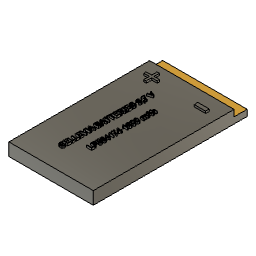
eBook_Reader (Autodesk Fusion 360 archive; units mm, degrees)
design "baterie"
Autodesk Fusion 360 part; units mm, degrees
sketch "Sketch1" plane through (0, 0, 0) normal (0, 0, 1) x (1, 0, 0)
  line L0 (0, 0) -> (42, 0)
  line L1 (42, 0) -> (42, 76.5)
  line L2 (42, 76.5) -> (0, 76.5)
  line L3 (0, 76.5) -> (0, 0)
  dimension "d1" = 42
  dimension "d2" = 76.5
  constraint horizontal L0
  constraint vertical L1
  constraint horizontal L2
  constraint vertical L3
  constraint coincident L0.start L3.end
  measures "d1" distance of L0.start L0.end
  measures "d2" distance of L0.start L2.end
extrude "Extrude1" add sketch "Sketch1" along normal blind 6.3
sketch "Sketch2" plane through (0, 0, 6.3) normal (0, 0, 1) x (-1, 0, 0)
  line L0 (0, -76.5) -> (0, 0)
  line L1 (0, 0) -> (-42, 0)
  line L2 (-42, 0) -> (-42, -76.5)
  line L3 (-42, -76.5) -> (0, -76.5)
  line L4 (0, -70) -> (-42, -70)
  constraint coincident L0 L4.start
  constraint coincident L2 L4.end
  constraint perpendicular L2 L4
extrude "Extrude2" cut sketch "Sketch2" against normal blind 3.2 contours L0 L2 L3 L4
sketch "Sketch3" plane through (0, 0, 6.3) normal (0, 0, 1) x (-1, 0, 0)
  line L0 (-42, -70) -> (0, -70)
  line L1 (0, -70) -> (0, 0)
  line L2 (0, 0) -> (-42, 0)
  line L3 (-42, 0) -> (-42, -70)
  line L4 (-5, -58) -> (-14, -58) construction
  line L5 (-14, -58) -> (-14, -66) construction
  line L6 (-14, -66) -> (-5, -66) construction
  line L7 (-5, -66) -> (-5, -58) construction
  dimension "d7" = 10
  text T0 "+\n" font "Arial" height 10 align left top in box 9 x 8 at (-5, -58) x (-1, 0) y (0, -1) spacing 1 kerned
extrude "Extrude3" add sketch "Sketch3" along normal blind 1 text T0
sketch "Sketch4" plane through (0, 0, 6.3) normal (0, 0, 1) x (-1, 0, 0)
  line L0 (-7.7217, -59.3902) -> (-7.7217, -62.1323)
  line L1 (-7.7217, -62.1323) -> (-5, -62.1323)
  line L2 (-5, -62.1323) -> (-5, -63.2783)
  line L3 (-5, -63.2783) -> (-7.7217, -63.2783)
  line L4 (-7.7217, -63.2783) -> (-7.7217, -66)
  line L5 (-7.7217, -66) -> (-8.8813, -66)
  line L6 (-8.8813, -66) -> (-8.8813, -63.2783)
  line L7 (-8.8813, -63.2783) -> (-11.603, -63.2783)
  line L8 (-11.603, -63.2783) -> (-11.603, -62.1323)
  line L9 (-11.603, -62.1323) -> (-8.8813, -62.1323)
  line L10 (-8.8813, -62.1323) -> (-8.8813, -59.3902)
  line L11 (-8.8813, -59.3902) -> (-7.7217, -59.3902)
  line L12 (-42, -70) -> (0, -70)
  line L13 (0, -70) -> (0, 0)
  line L14 (0, 0) -> (-42, 0)
  line L15 (-42, 0) -> (-42, -70)
  line L16 (-31, -59) -> (-37, -59) construction
  line L17 (-37, -59) -> (-37, -63) construction
  line L18 (-37, -63) -> (-31, -63) construction
  line L19 (-31, -63) -> (-31, -59) construction
  dimension "d10" = 15
  text T0 "-" font "Arial" height 15 align left top in box 6 x 4 at (-31, -59) x (-1, 0) y (0, -1) spacing 1 kerned
extrude "Extrude4" add sketch "Sketch4" along normal blind 1 text T0
sketch "Sketch5" plane through (0, 0, 6.3) normal (0, 0, 1) x (-1, 0, 0)
  line L0 (-31, -61.148) -> (-31, -63)
  line L1 (-31, -63) -> (-36.6583, -63)
  line L2 (-36.6583, -63) -> (-36.6583, -61.148)
  line L3 (-36.6583, -61.148) -> (-31, -61.148)
  line L4 (-7.7217, -59.3902) -> (-7.7217, -62.1323)
  line L5 (-7.7217, -62.1323) -> (-5, -62.1323)
  line L6 (-5, -62.1323) -> (-5, -63.2783)
  line L7 (-5, -63.2783) -> (-7.7217, -63.2783)
  line L8 (-7.7217, -63.2783) -> (-7.7217, -66)
  line L9 (-7.7217, -66) -> (-8.8813, -66)
  line L10 (-8.8813, -66) -> (-8.8813, -63.2783)
  line L11 (-8.8813, -63.2783) -> (-11.603, -63.2783)
  line L12 (-11.603, -63.2783) -> (-11.603, -62.1323)
  line L13 (-11.603, -62.1323) -> (-8.8813, -62.1323)
  line L14 (-8.8813, -62.1323) -> (-8.8813, -59.3902)
  line L15 (-8.8813, -59.3902) -> (-7.7217, -59.3902)
  line L16 (-42, -70) -> (0, -70)
  line L17 (0, -70) -> (0, 0)
  line L18 (0, 0) -> (-42, 0)
  line L19 (-42, 0) -> (-42, -70)
  line L20 (-29.8057, -5.0482) -> (-30.6288, -60.9755) construction
  line L21 (-30.6288, -60.9755) -> (-14.6018, -61.2113) construction
  line L22 (-14.6018, -61.2113) -> (-13.7788, -5.2841) construction
  line L23 (-13.7788, -5.2841) -> (-29.8057, -5.0482) construction
  dimension "d13" = 2.5
  text T0 "CELLEVIA BATTERIES 3,7 V\n\nLP584174 1800 mAh" font "Arial" height 2.5 align centre top in box 55.9333 x 16.0287 at (-29.8057, -5.0482) x (-0.014714, -0.999892) y (0.999892, -0.014714) spacing 1
extrude "Extrude5" add sketch "Sketch5" along normal blind 1 text T0

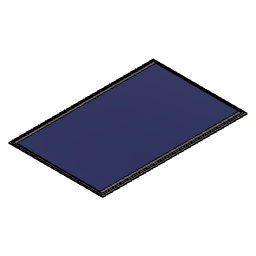
design "display"
Autodesk Fusion 360 part; units mm, degrees
sketch "Sketch1" plane through (0, 0, 0) normal (0, 0, 1) x (1, 0, 0)
  line L0 (0, 0) -> (111.2, 0)
  line L1 (111.2, 0) -> (111.2, 170.2)
  line L2 (111.2, 170.2) -> (0, 170.2)
  line L3 (0, 170.2) -> (0, 0)
  dimension "d1" = 111.2
  dimension "d2" = 170.2
  constraint horizontal L0
  constraint vertical L1
  constraint horizontal L2
  constraint vertical L3
  constraint coincident L0.start L3.end
  measures "d1" distance of L0.start L0.end
  measures "d2" distance of L0.start L2.end
extrude "Extrude1" add sketch "Sketch1" along normal blind 0.7
sketch "Sketch2" plane through (0, 0, 0.7) normal (0, 0, 1) x (-1, 0, 0)
  line L0 (0, -170.2) -> (0, 0)
  line L1 (0, 0) -> (-111.2, 0)
  line L2 (-111.2, 0) -> (-111.2, -170.2)
  line L3 (-111.2, -170.2) -> (0, -170.2)
  line L4 (-109.145, -1.2) -> (-2.055, -1.2)
  line L5 (-2.055, -1.2) -> (-2.055, -169)
  line L6 (-2.055, -169) -> (-109.145, -169)
  line L7 (-109.145, -169) -> (-109.145, -1.2)
  line L8 (-109.145, -1.2) -> (-2.055, -169) construction
  line L9 (-2.055, -1.2) -> (-109.145, -169) construction
  point P0 (-55.6, -85.1)
  dimension "d5" = 107.09
  dimension "d6" = 167.8
  constraint horizontal L4
  constraint perpendicular L4 L5
  constraint parallel L4 L6
  constraint parallel L5 L7
  constraint coincident L8 P0
  constraint coincident L9 P0
  measures "d5" distance of L5.end L6.end
  measures "d6" distance of L4.end L5.end
extrude "Extrude2" add sketch "Sketch2" along normal blind 0.55 contours L4 L5 L6 L7
sketch "Sketch3" plane through (0, 0, 1.25) normal (0, 0, 1) x (-1, 0, 0)
  line L0 (-109.145, -169) -> (-2.055, -169)
  line L1 (-2.055, -169) -> (-2.055, -1.2)
  line L2 (-2.055, -1.2) -> (-109.145, -1.2)
  line L3 (-109.145, -1.2) -> (-109.145, -169)
  line L4 (-107.645, -167.5) -> (-3.555, -167.5)
  line L5 (-3.555, -167.5) -> (-3.555, -2.7)
  line L6 (-3.555, -2.7) -> (-107.645, -2.7)
  line L7 (-107.645, -2.7) -> (-107.645, -167.5)
  line L8 (-107.645, -167.5) -> (-3.555, -2.7) construction
  line L9 (-3.555, -167.5) -> (-107.645, -2.7) construction
  point P0 (-55.6, -85.1)
  dimension "d9" = 104.09
  dimension "d10" = 164.8
  constraint horizontal L4
  constraint perpendicular L4 L5
  constraint parallel L4 L6
  constraint parallel L5 L7
  constraint coincident L8 P0
  constraint coincident L9 P0
  measures "d9" distance of L5.end L6.end
  measures "d10" distance of L4.end L5.end
extrude "Extrude3" add sketch "Sketch3" along normal blind 0.55 contours L4 L5 L6 L7
sketch "Sketch4" plane through (0, 0, 1.8) normal (0, 0, 1) x (-1, 0, 0)
  line L0 (-107.645, -2.7) -> (-107.645, -167.5)
  line L1 (-107.645, -167.5) -> (-3.555, -167.5)
  line L2 (-3.555, -167.5) -> (-3.555, -2.7)
  line L3 (-3.555, -2.7) -> (-107.645, -2.7)
  line L4 (-6.64, -3.5) -> (-104.56, -3.5)
  line L5 (-104.56, -3.5) -> (-104.56, -166.7)
  line L6 (-104.56, -166.7) -> (-6.64, -166.7)
  line L7 (-6.64, -166.7) -> (-6.64, -3.5)
  line L8 (-6.64, -3.5) -> (-104.56, -166.7) construction
  line L9 (-104.56, -3.5) -> (-6.64, -166.7) construction
  point P0 (-55.6, -85.1)
  dimension "d13" = 97.92
  dimension "d14" = 163.2
  constraint horizontal L4
  constraint perpendicular L4 L5
  constraint parallel L4 L6
  constraint parallel L5 L7
  constraint coincident L8 P0
  constraint coincident L9 P0
  measures "d13" distance of L5.end L6.end
  measures "d14" distance of L4.end L5.end
extrude "Extrude4" add sketch "Sketch4" along normal blind 0.01 contours L4 L5 L6 L7
extrude "Extrude5" cut 1 faces at (0, 113.4667, 0.2333) along direction (1, 0, 0) blind 0.353
extrude "Extrude6" cut 1 faces at (71.92, 57.9, 1.81) along direction (0, 0, -1) blind 0.01
extrude "Extrude7" cut 1 faces at (72.9483, 57.6333, 1.8) along direction (0, 0, -1) blind 0.55
extrude "Extrude8" cut 1 faces at (73.4483, 57.1333, 1.25) along direction (0, 0, -1) blind 0.31
sketch "Sketch5" plane through (0, 0, 0.94) normal (0, 0, 1) x (-1, 0, 0)
  line L0 (-109.145, -169) -> (-2.055, -169)
  line L1 (-2.055, -169) -> (-2.055, -1.2)
  line L2 (-2.055, -1.2) -> (-109.145, -1.2)
  line L3 (-109.145, -1.2) -> (-109.145, -169)
  line L4 (-3.555, -2.7) -> (-107.645, -2.7)
  line L5 (-107.645, -2.7) -> (-107.645, -167.5)
  line L6 (-107.645, -167.5) -> (-3.555, -167.5)
  line L7 (-3.555, -167.5) -> (-3.555, -2.7)
  line L8 (-3.555, -2.7) -> (-107.645, -167.5) construction
  line L9 (-107.645, -2.7) -> (-3.555, -167.5) construction
  point P0 (-55.6, -85.1)
  dimension "d25" = 104.09
  dimension "d26" = 164.8
  constraint horizontal L4
  constraint perpendicular L4 L5
  constraint parallel L4 L6
  constraint parallel L5 L7
  constraint coincident L8 P0
  constraint coincident L9 P0
  measures "d25" distance of L5.end L6.end
  measures "d26" distance of L4.end L5.end
extrude "Extrude9" add sketch "Sketch5" along normal blind 0.24 contours L4 L5 L6 L7
sketch "Sketch6" plane through (0, 0, 1.18) normal (0, 0, 1) x (-1, 0, 0)
  line L0 (-3.555, -167.5) -> (-3.555, -2.7)
  line L1 (-3.555, -2.7) -> (-107.645, -2.7)
  line L2 (-107.645, -2.7) -> (-107.645, -167.5)
  line L3 (-107.645, -167.5) -> (-3.555, -167.5)
  line L4 (-6.64, -166.7) -> (-104.56, -166.7)
  line L5 (-104.56, -166.7) -> (-104.56, -3.5)
  line L6 (-104.56, -3.5) -> (-6.64, -3.5)
  line L7 (-6.64, -3.5) -> (-6.64, -166.7)
  line L8 (-6.64, -166.7) -> (-104.56, -3.5) construction
  line L9 (-104.56, -166.7) -> (-6.64, -3.5) construction
  point P0 (-55.6, -85.1)
  dimension "d29" = 97.92
  dimension "d30" = 163.2
  constraint horizontal L4
  constraint perpendicular L4 L5
  constraint parallel L4 L6
  constraint parallel L5 L7
  constraint coincident L8 P0
  constraint coincident L9 P0
  measures "d29" distance of L5.end L6.end
  measures "d30" distance of L4.end L5.end
extrude "Extrude10" add sketch "Sketch6" along normal blind 0.01 contours L4 L5 L6 L7
extrude "Extrude11" cut 1 faces at (0.353, 113.4667, 0.2333) along direction (1, 0, 0) blind 0.266
